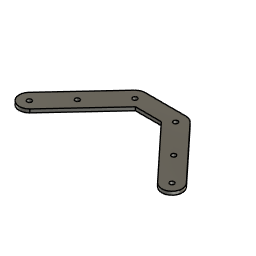
GearPlate v5 (Autodesk Fusion 360 design; units mm, degrees)
Autodesk Fusion 360 part; units mm, degrees
sketch "Sketch1" plane through (0, 0, 0) normal (0, 0, 1) x (1, 0, 0)
  circle A0 centre (0, 0) radius 3.275
  circle A1 centre (210, 0) radius 3.275
  circle A2 centre (0, 0) radius 15
  circle A3 centre (210, 0) radius 15
  line L0 (0, 15) -> (210, 15)
  line L1 (0, -15) -> (210, -15)
  circle A4 centre (0, 0) radius 20 construction
  circle A5 centre (210, 0) radius 20 construction
  circle A6 centre (75, 80.4674) radius 3.275
  circle A7 centre (135, 80.4674) radius 3.275
  circle A8 centre (75, 80.4674) radius 15
  circle A9 centre (135, 80.4674) radius 15
  line L2 (-10.9728, 10.2273) -> (64.0272, 90.6947)
  line L3 (75, 95.4674) -> (135, 95.4674)
  line L4 (145.9728, 90.6947) -> (220.9728, 10.2273)
  circle A10 centre (34.0909, 36.5761) radius 30 construction
  circle A11 centre (75, 80.4674) radius 30 construction
  circle A12 centre (175.9091, 36.5761) radius 30 construction
  circle A13 centre (135, 80.4674) radius 30 construction
  line L5 (0, 0) -> (75, 80.4674) construction
  circle A14 centre (34.0909, 36.5761) radius 3.275
  circle A15 centre (175.9091, 36.5761) radius 3.275
  line L6 (10.9728, -10.2273) -> (85.9728, 70.2401)
  line L7 (199.0272, -10.2273) -> (124.0272, 70.2401)
  line L8 (85.9728, 70.2401) -> (124.0272, 70.2401)
  dimension "d2" = 6.55
  dimension "d3" = 6.55
  dimension "d4" = 210
  dimension "d6" = 30
  dimension "d7" = 30
  dimension "d10" = 40
  dimension "d11" = 40
  dimension "d14" = 6.55
  dimension "d15" = 6.55
  dimension "d16" = 30
  dimension "d17" = 30
  dimension "d20" = 60
  dimension "d21" = 60
  dimension "d22" = 60
  dimension "d23" = 60
  dimension "d24" = 6.55
  dimension "d25" = 6.55
  constraint coincident A0.centre A2.centre
  constraint horizontal A0.centre A1.centre
  constraint concentric A0 A2
  constraint concentric A1 A3
  constraint coincident A2 L0.start
  constraint coincident A3 L0.end
  constraint tangent A3 L0
  constraint horizontal L0
  constraint coincident A2 L1.start
  constraint coincident A3 L1.end
  constraint tangent A3 L1
  constraint parallel L0 L1
  constraint concentric A0 A4
  constraint concentric A1 A5
  constraint concentric A7 A9
  constraint coincident A2 L2.start
  constraint coincident A8 L2.end
  constraint tangent A8 L2
  constraint coincident A8 L3.start
  constraint coincident A9 L3.end
  constraint tangent A9 L3
  constraint coincident A9 L4.start
  constraint coincident A3 L4.end
  constraint tangent A3 L4
  constraint tangent A9 L4
  constraint tangent A2 L2
  constraint tangent A8 L3
  constraint concentric A6 A8
  constraint tangent A4 A10
  constraint tangent A5 A12
  constraint tangent A12 A13
  constraint tangent A11 A13
  constraint tangent A10 A11
  constraint horizontal A6.centre A7.centre
  constraint horizontal A10.centre A12.centre
  constraint coincident A6.centre A8.centre
  constraint coincident A10.centre L5
  constraint coincident A7.centre A9.centre
  constraint concentric A10 A14
  constraint concentric A12 A15
  constraint coincident A2 L6.start
  constraint coincident A8 L6.end
  constraint tangent A8 L6
  constraint coincident A3 L7.start
  constraint coincident A9 L7.end
  constraint tangent A9 L7
  constraint tangent A2 L6
  constraint tangent A3 L7
  measures "d2" diameter of A0
  measures "d3" diameter of A1
  measures "d4" distance of A0.centre A1.centre
  measures "d6" diameter of A2
  measures "d7" diameter of A3
  measures "d10" diameter of A4
  measures "d11" diameter of A5
  measures "d14" diameter of A6
  measures "d15" diameter of A7
  measures "d16" diameter of A8
  measures "d17" diameter of A9
  measures "d20" diameter of A10
  measures "d21" diameter of A11
  measures "d22" diameter of A12
  measures "d23" diameter of A13
  measures "d24" diameter of A14
  measures "d25" diameter of A15
extrude "Extrude1" add sketch "Sketch1" along normal blind 5 contours A2 | A2 L0 L6 | A2 L0 A8 L2 L6 | A8 | A3 L0 A9 L4 L7 | A3 L0 L7 | A8 A9 L3 L8 | A3 | A9
equation "SlipGearNominal = 209.5 mm"
equation "d4 = SlipGearNominal + SlipGearOffset"
equation "SlipGearOffset = 0.5 mm"
